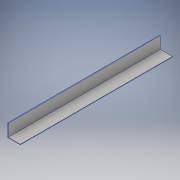
# Autodesk Inventor part: Aluminum Angle Channel-01
Saved by Autodesk Inventor 2017.3 (Build 213256000, 256)
## iProperties
Created: 2019-04-27
Part Number: Aluminum Angle Channel-01
Material: Aluminum 6061
Document SubType Name: Modeling
Designer: guberti
Density: 2.7 g/cm^3
Appearance: Aluminum - Flat
Author: guberti
Autodesk Inventor part; units mm, degrees
ref_plane "YZ Plane" through (0, 0, 0) normal (1, 0, 0) x (0, 1, 0)
ref_plane "XZ Plane" through (0, 0, 0) normal (0, 1, 0) x (-1, 0, 0)
ref_plane "XY Plane" through (0, 0, 0) normal (0, 0, 1) x (1, 0, 0)
sketch "Sketch1" plane through (0, 0, 0) normal (0, 0, 1) x (1, 0, 0)
  line L0 (0, 0) -> (38.1, 0)
  line L1 (38.1, 0) -> (38.1, 1.5875)
  line L2 (38.1, 1.5875) -> (1.5875, 1.5875)
  line L3 (1.5875, 1.5875) -> (1.5875, 38.1)
  line L4 (1.5875, 38.1) -> (0, 38.1)
  line L5 (0, 38.1) -> (0, 0)
  dimension "leglength" = 38.1
  dimension "thickness" = 1.5875
  dimension "d2" = 36.5125
  dimension "d3" = 36.5125
  dimension "d4" = 1.5875
  constraints: 12 end point, 4 perpendicular, 1 horizontal
  measures "leglength" distance of L0.start L0.end
  measures "thickness" distance of L0.end L1.end
  measures "d2" distance of L1.end L2.end
  measures "d3" distance of L2.end L3.end
  measures "d4" distance of L3.end L4.end
extrude "Extrusion1" add sketch "Sketch1" along normal blind 457.2
equation "\"d2\" = leglength - thickness"
equation "\"d3\" = leglength - thickness"
equation "\"d4\" = thickness"
equation "\"d5\" = length"
equation "\"length\" = 457.2"
body "Solid1"
